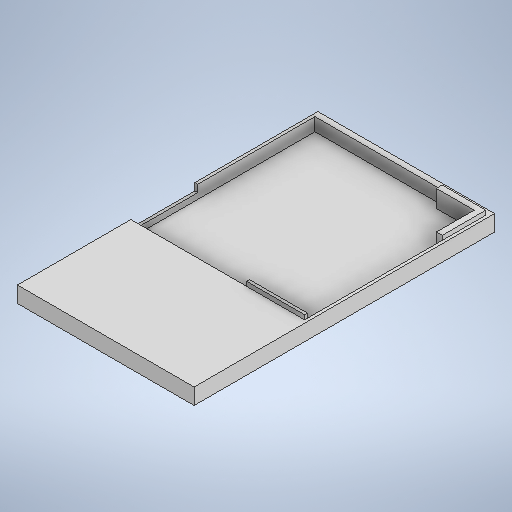
# Autodesk Inventor part: Lid bottom
Saved by Autodesk Inventor 2025.2 (Build 292293000, 293)
## iProperties
Created: 2025-04-04
Part Number: Lid bottom
Material: Generic
Document SubType Name: Modeling
Designer: joaki
Density: 1 g/cm^3
Appearance: Default
Author: joaki
Autodesk Inventor part; units mm, degrees
ref_plane "YZ Plane" through (0, 0, 0) normal (1, 0, 0) x (0, 1, 0)
ref_plane "XZ Plane" through (0, 0, 0) normal (0, 1, 0) x (-1, 0, 0)
ref_plane "XY Plane" through (0, 0, 0) normal (0, 0, 1) x (1, 0, 0)
sketch "Sketch1" plane through (0, 0, 0) normal (0, 1, 0) x (-1, 0, 0)
  line L0 (32.9806, 40.5565) -> (-27.7594, 40.5565)
  line L1 (-27.7594, 40.5565) -> (-27.7594, -62.7415)
  line L2 (-27.7594, -62.7415) -> (32.9806, -62.7415)
  line L3 (32.9806, -62.7415) -> (32.9806, 40.5565)
  point P0 (0, 0)
  dimension "d0" = 60.74
  dimension "d1" = 103.298
  constraints: 8 end point, 2 parallel, 1 horizontal, 1 perpendicular
  measures "d0" distance of L1.end L2.end
  measures "d1" distance between parallel lines of L2 L0
extrude "Extrusion1" add sketch "Sketch1" along normal blind 1
sketch "Sketch2" plane through (0, 1, 0) normal (0, 1, 0) x (1, 0, 0)
  line L0 (-32.9806, 62.7415) -> (-32.9806, -40.5565) projected
  line L1 (27.7594, -40.5565) -> (27.7594, 62.7415) projected
  line L2 (-32.9806, -40.5565) -> (27.7594, -40.5565)
  line L3 (27.7594, -40.5565) -> (27.7594, -1.5565)
  line L4 (27.7594, -1.5565) -> (-32.9806, -1.5565)
  line L5 (-32.9806, -1.5565) -> (-32.9806, -40.5565)
  point P0 (0, 0)
  point P1 (-32.9806, -1.5565)
  dimension "d4" = 39
  constraints: 8 end point, 2 parallel, 1 horizontal, 1 perpendicular, 1 point on line
  measures "d4" distance between parallel lines of L4 L2
extrude "Extrusion2" add sketch "Sketch2" along normal blind 4.5
sketch "Sketch3" plane through (0, 1, 0) normal (0, 1, 0) x (1, 0, 0)
  line L0 (27.7594, -1.5565) -> (-32.9806, -1.5565) projected
  line L1 (27.7594, 62.7415) -> (-32.9806, 62.7415) projected
  line L2 (-32.9806, -1.5565) -> (-31.9806, -1.5565)
  line L3 (-31.9806, -1.5565) -> (-31.9806, 62.7415)
  line L4 (-31.9806, 62.7415) -> (-32.9806, 62.7415)
  line L5 (-32.9806, 62.7415) -> (-32.9806, -1.5565)
  line L6 (-31.9806, 62.7415) -> (27.7594, 62.7415)
  line L7 (27.7594, 62.7415) -> (27.7594, 60.7415)
  line L8 (27.7594, 60.7415) -> (-31.9806, 60.7415)
  line L9 (-31.9806, 60.7415) -> (-31.9806, 62.7415)
  line L10 (27.7594, -40.5565) -> (27.7594, 62.7415) projected
  line L11 (27.7594, -1.5565) -> (26.7594, -1.5565)
  line L12 (26.7594, -1.5565) -> (26.7594, 60.7415)
  line L13 (26.7594, 60.7415) -> (27.7594, 60.7415)
  line L14 (27.7594, 60.7415) -> (27.7594, -1.5565)
  line L15 (-32.9806, -1.5565) -> (-31.9806, -1.5565)
  line L16 (-31.9806, -1.5565) -> (-31.9806, 20.4435)
  line L17 (-31.9806, 20.4435) -> (-32.9806, 20.4435)
  line L18 (-32.9806, 20.4435) -> (-32.9806, -1.5565)
  point P0 (0, 0)
  point P1 (27.2594, -1.5565)
  point P2 (-31.9806, 60.7415)
  point P3 (-32.4806, -1.5565)
  point P4 (-32.4806, 20.4435)
  dimension "d7" = 1
  dimension "d8" = 2
  dimension "d9" = 1
  dimension "d10" = 0
  dimension "d13" = 22
  constraints: 32 end point, 8 parallel, 4 horizontal, 4 perpendicular, 4 point on line, 3 midpoint
  measures "d7" distance between parallel lines of L5 L3
  measures "d8" distance between parallel lines of L1 L8
  measures "d9" distance between parallel lines of L14 L12
  measures "d10" distance from line of L0 point (27.259, -1.557)
  measures "d13" distance of point (-32.481, -1.557) point (-32.481, 20.443)
extrude "Extrusion3" add sketch "Sketch3" along normal blind 4.5 contours L0 L12 L8 L10 | L8 L3 L1 L7 | L17 L5 L1 L3
sketch "Sketch4" plane through (0, 1, 0) normal (0, 1, 0) x (1, 0, 0)
  line L0 (-32.9806, 62.7415) -> (-32.9806, -40.5565) projected
  line L1 (-31.9806, 20.4435) -> (-32.9806, 20.4435)
  line L2 (-32.9806, 20.4435) -> (-32.9806, -2.617)
  line L3 (-32.9806, -2.617) -> (-31.9806, -2.617)
  line L4 (-31.9806, -2.617) -> (-31.9806, 20.4435)
  point P0 (0, 0)
  constraints: 8 end point, 2 parallel, 1 horizontal, 1 perpendicular, 1 point on line
extrude "Extrusion4" add sketch "Sketch4" along normal blind 2
sketch "Sketch5" plane through (0, 1, 0) normal (0, 1, 0) x (1, 0, 0)
  line L0 (26.7594, 60.7415) -> (26.7594, -1.5565) projected
  line L1 (26.7594, 60.7415) -> (11.7594, 60.7415)
  line L2 (11.7594, 60.7415) -> (11.7594, 58.7415)
  line L3 (11.7594, 58.7415) -> (26.7594, 58.7415)
  line L4 (26.7594, 58.7415) -> (26.7594, 60.7415)
  line L5 (26.7594, 60.7415) -> (24.7594, 60.7415)
  line L6 (24.7594, 60.7415) -> (24.7594, 45.7415)
  line L7 (24.7594, 45.7415) -> (26.7594, 45.7415)
  line L8 (26.7594, 45.7415) -> (26.7594, 60.7415)
  line L9 (26.7594, -1.5565) -> (6.7594, -1.5565)
  line L10 (6.7594, -1.5565) -> (6.7594, -0.5565)
  line L11 (6.7594, -0.5565) -> (26.7594, -0.5565)
  line L12 (26.7594, -0.5565) -> (26.7594, -1.5565)
  point P0 (0, 0)
  point P1 (26.7594, 59.7415)
  point P2 (11.7594, 59.7415)
  point P3 (25.7594, 45.7415)
  point P4 (25.7594, 60.7415)
  point P5 (26.7594, -1.0565)
  point P6 (6.7594, -1.0565)
  point P7 (24.7594, 58.7415)
  dimension "d16" = 2
  dimension "d17" = 15
  dimension "d18" = 2
  dimension "d19" = 15
  dimension "d20" = 1
  dimension "d21" = 20
  constraints: 24 end point, 6 midpoint, 6 parallel, 3 horizontal, 3 perpendicular
  measures "d16" distance between parallel lines of L1 L3
  measures "d17" distance of point (26.759, 59.741) point (11.759, 59.741)
  measures "d18" distance between parallel lines of L0 L6
  measures "d19" distance of point (25.759, 45.741) point (25.759, 60.741)
  measures "d20" distance between parallel lines of L11 L9
  measures "d21" distance of point (26.759, -1.057) point (6.759, -1.057)
extrude "Extrusion5" add sketch "Sketch5" along normal blind 6
body "Solid1"
